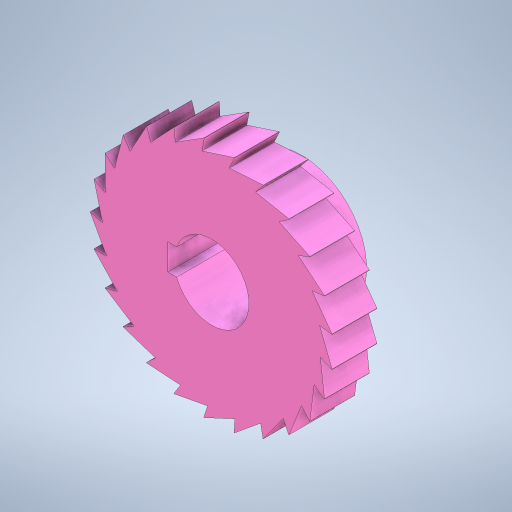
# Autodesk Inventor part: Pieza Propia Ensamblaje - Alison
Saved by Autodesk Inventor 2024 (Build 280153000, 153)
## iProperties
Created: 2024-03-29
Part Number: Pieza Propia Ensamblaje - Alison
Material: Genérico
Document SubType Name: Modeling
Designer: Alison
Density: 1 g/cm^3
Appearance: Valor por defecto
Author: Alison
Autodesk Inventor part; units mm, degrees
ref_plane "YZ Plane" through (0, 0, 0) normal (1, 0, 0) x (0, 1, 0)
ref_plane "XZ Plane" through (0, 0, 0) normal (0, 1, 0) x (-1, 0, 0)
ref_plane "XY Plane" through (0, 0, 0) normal (0, 0, 1) x (1, 0, 0)
sketch "Boceto1" plane through (0, 0, 0) normal (0, 0, 1) x (1, 0, 0)
  circle A0 centre (0, 0) radius 32.5
  circle A1 centre (0, 0) radius 10
  line L0 (0, -32.5) -> (0, 0) construction
  line L1 (0, -32.5) -> (-9.058, -23.9422)
  line L2 (-9.058, -23.9422) -> (-10.8513, -30.6349)
  dimension "d0" = 65
  dimension "d1" = 20
  dimension "d4" = 15
  constraints: 6 end point, 2 centre point, 2 coincident, 2 point on circle, 1 vertical
  measures "d0" diameter of A0
  measures "d1" diameter of A1
  measures "d4" angle of L2 L0
extrude "Extrusión1" add sketch "Boceto1" along normal blind 12
sketch "Boceto2" plane through (0, 0, 12) normal (0, 0, 1) x (1, 0, 0)
  line L0 (-32.5, 0) -> (0, 0) construction
  line L1 (-32.5, 0) -> (-28.1293, -8)
  line L2 (-28.1293, -8) -> (-31.5, -8)
  circle A0 centre (0, 0) radius 29.2448 construction
  arc A1 (-32.5, 0) -> (-31.5, -8) centre (0, 0) ccw construction
  arc A2 (-32.5, 0) -> (-31.5, -8) centre (0, 0) ccw construction
  circle A3 centre (0, 0) radius 10 projected
  arc A4 (-32.5, 0) -> (-31.5, -8) centre (0, 0) ccw
  dimension "d5" = 8
  dimension "d7" = 8
  dimension "d22" = 20
  constraints: 6 end point, 6 point on circle, 4 coincident, 3 centre point, 2 horizontal, 1 concentric, 3 other
  measures "d5" distance between parallel lines of L2 L0
  measures "d7" vertical distance of L0.start L1.end
  measures "d22" diameter of A3
extrude "Extrusión2" cut sketch "Boceto2" against normal blind 12 contours L1 L2 A4
pattern_circular "Patrón circular1" count 25 over 360 about axis through (0, 0, -10) along (0, 0, 1) of "Extrusión2"
sketch "Boceto3" plane through (0, 0, 0) normal (0, 0, -1) x (-1, 0, 0)
  circle A0 centre (0, 0) radius 17.5
  circle A1 centre (0, 0) radius 10
  dimension "d13" = 35
  dimension "d23" = 20
  constraints: 2 centre point, 2 coincident
  measures "d13" diameter of A0
  measures "d23" diameter of A1
extrude "Extrusión3" add sketch "Boceto3" along normal blind 12
sketch "Boceto5" plane through (0, 0, -12) normal (0, 0, -1) x (-1, 0, 0)
  circle A0 centre (0, 0) radius 10 projected
  line L0 (11.725, -3.5) -> (8.275, 3.5) construction
  line L1 (8.275, -3.5) -> (11.725, 3.5) construction
  line L2 (9.3675, 3.5) -> (11.725, 3.5)
  line L3 (11.725, -3.5) -> (9.3675, -3.5)
  arc A1 (9.3675, 3.5) -> (9.3675, -3.5) centre (0, 0) ccw
  line L4 (11.725, 3.5) -> (11.725, -3.5)
  dimension "d24" = 3.45
  dimension "d25" = 7
  constraints: 10 end point, 4 point on circle, 1 centre point, 1 coincident, 1 concentric, 1 perpendicular
  measures "d24" distance of L0.end L1.end
  measures "d25" distance of L1.start L0.end
extrude "Extrusión4" cut sketch "Boceto5" against normal blind 24 contours A0 L2 L4 L3
